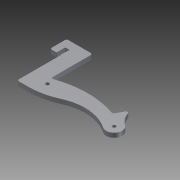
# Autodesk Inventor part: soporte bobina nuevo
Saved by Autodesk Inventor 2012 SP1 (Build 160190100, 190)
## iProperties
Created: 2015-03-15
Part Number: soporte bobina nuevo
Material: Default
Document SubType Name: Modeling
Designer: Laser router cnc
Density: 1 g/cm^3
Author: Laser router cnc
Autodesk Inventor part; units mm, degrees
ref_plane "YZ Plane" through (0, 0, 0) normal (1, 0, 0) x (0, 1, 0)
ref_plane "XZ Plane" through (0, 0, 0) normal (0, 1, 0) x (-1, 0, 0)
ref_plane "XY Plane" through (0, 0, 0) normal (0, 0, 1) x (1, 0, 0)
sketch "Boceto1" plane through (0, 0, 0) normal (0, 0, 1) x (1, 0, 0)
  line L0 (0, 26.9924) -> (5, 26.9924)
  arc A0 (5, 26.9924) -> (5.5, 27.4924) centre (5, 27.4924) ccw
  line L1 (5.5, 27.4924) -> (5.5, 36.4924)
  arc A1 (6, 36.9924) -> (5.5, 36.4924) centre (6, 36.4924) ccw
  line L2 (6, 36.9924) -> (9.9731, 36.9924)
  arc A2 (10.4724, 36.4662) -> (9.9731, 36.9924) centre (9.9731, 36.4924) ccw
  line L3 (10.4724, 36.4662) -> (10.0035, 27.5185)
  arc A3 (10.0035, 27.5185) -> (10.5028, 26.9924) centre (10.5028, 27.4924) ccw
  arc A4 (23, -23.0504) -> (54.0922, -16.3077) centre (23, 52.0085) ccw
  arc A5 (106.311, -20.6517) -> (54.0922, -16.3077) centre (76.3195, -65.146) ccw
  arc A6 (106.311, -20.6517) -> (116.3303, -5.6981) centre (111.3414, -13.1888) ccw
  arc A7 (106.3579, 7.7696) -> (116.3303, -5.6981) centre (130.0298, 14.8719) ccw
  arc A8 (106.3579, 7.7696) -> (102.827, 7.7277) centre (104.6036, 6.8117) ccw
  line L4 (102.827, 7.7277) -> (98.8026, -0.0781)
  arc A9 (96.3676, -1.0494) -> (98.8026, -0.0781) centre (97.026, 0.8379) ccw
  arc A10 (96.3676, -1.0494) -> (30.1711, -1.1614) centre (63.429, -95.4689) ccw
  line L5 (13.5421, 45.9924) -> (0, 45.9924)
  arc A11 (0, 45.9924) -> (-1.9988, 43.9936) centre (0, 43.9936) ccw
  line L6 (-1.9988, 43.9936) -> (-1.9988, 28.9912)
  arc A12 (-1.9988, 28.9912) -> (0, 26.9924) centre (0, 28.9912) ccw
  circle A13 centre (111.3414, -13.1888) radius 1.9988
  circle A14 centre (31.3414, -9.1385) radius 1.9988
  line L7 (10.5028, 26.9924) -> (10.5028, -23.0504)
  line L8 (23, -23.0504) -> (13.5421, -23.0504)
  line L9 (13.5421, 45.9924) -> (27.5683, 45.9924)
  line L10 (27.5683, 45.9924) -> (27.5683, -2)
  arc A15 (27.5683, -2) -> (30.1711, -1.1614) centre (13.5421, 45.9924) ccw
  line L11 (13.5421, -23.0504) -> (10.5028, -23.0504)
  point P0 (0, 0)
  constraints: 28 point on circle, 24 end point, 19 tangent, 16 centre point, 8 equal radius, 5 perpendicular, 4 parallel, 1 concentric
extrude "Extrusión2" add sketch "Boceto1" along normal blind 5
fillet "Empalme1" radius 2 3 edges at (10.5028, -23.0504, 2.5) (27.5683, 45.9924, 2.5) (27.5683, -2, 2.5)
